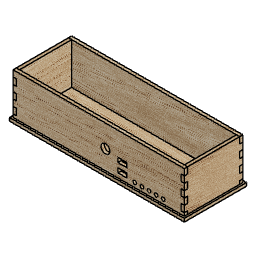
wood chassis (Autodesk Fusion 360 design; units mm, degrees)
Autodesk Fusion 360 part; units mm, degrees
sketch "base" plane through (0, 0, 0) normal (0, 0, 1) x (1, 0, 0) in component "base"
  line L0 (0, 0) -> (192.2, 0)
  line L1 (192.2, 0) -> (192.2, 65.7)
  line L2 (192.2, 65.7) -> (0, 65.7)
  line L3 (0, 65.7) -> (0, 0)
  line L4 (192.2, 32.85) -> (0, 32.85) construction
  line L5 (96.1, 65.7) -> (96.1, 0) construction
  line L6 (-2, 67.7) -> (194.2, 67.7)
  line L7 (194.2, 67.7) -> (194.2, -2)
  line L8 (194.2, -2) -> (-2, -2)
  line L9 (-2, -2) -> (-2, 67.7)
  line L10 (-2, 67.7) -> (194.2, -2) construction
  line L11 (194.2, 67.7) -> (-2, -2) construction
  point P0 (96.1, 32.85)
  dimension "d14" = 192.2
  dimension "d15" = 65.7
  dimension "d16" = 2
  dimension "d17" = 2
  constraint horizontal L0
  constraint vertical L1
  constraint horizontal L2
  constraint vertical L3
  constraint coincident L0.start L3.end
  constraint midpoint L1 L4.start
  constraint midpoint L3 L4.end
  constraint midpoint L2 L5.start
  constraint midpoint L0 L5.end
  constraint horizontal L6
  constraint perpendicular L6 L7
  constraint parallel L6 L8
  constraint parallel L7 L9
  constraint coincident L10 P0
  constraint coincident L11 P0
  constraint midpoint L4 P0
  measures "d14" distance of L1.end L2.end
  measures "d15" distance of L0.end L1.end
  measures "d16" distance of L2 L6
  measures "d17" distance of L1 L7
extrude "Extrude1" add sketch "base" along normal blind 3.6 contours L0 L1 L2 L3 | L6 L7 L8 L9 makes body 1 in component "base"
sketch "lenghttabcut" plane through (0, 0, 3.6) normal (0, 0, 1) x (-1, 0, 0) in component "base"
  line L0 (2, 2) -> (-194.2, 2)
  line L1 (-194.2, 2) -> (-194.2, -67.7)
  line L2 (-194.2, -67.7) -> (2, -67.7)
  line L3 (2, -67.7) -> (2, 2)
  line L4 (-27.4571, -65.7) -> (-54.9143, -65.7)
  line L5 (-54.9143, -65.7) -> (-54.9143, -62.1)
  line L6 (-54.9143, -62.1) -> (-27.4571, -62.1)
  line L7 (-27.4571, -62.1) -> (-27.4571, -65.7)
  line L8 (-192.2, -65.7) -> (0, -65.7)
  line L9 (0, -65.7) -> (0, 0)
  dimension "d20" = 27.4571
  dimension "d21" = 27.4571
  dimension "d35" = 3.6
  constraint horizontal L4
  constraint vertical L5
  constraint horizontal L6
  constraint vertical L7
  constraint collinear L4 L8
  measures "d20" distance of L7 L9
  measures "d21" distance of L4.start L4.end
  measures "d35" distance of L4.start L6.end
extrude "Extrude2" cut sketch "lenghttabcut" against normal blind 3.6 contours L4 L5 L6 L7 L8 bodies 1 in component "base"
pattern_linear "R-Pattern1" count 3 spacing 54.9143 along (1, 0, 0) of "Extrude2" in component "base"
ref_plane "WorkPlane1" through (96.1, 65.7, 1.8) normal (0, 1, 0) x (-1, 0, 0) in component "back"
sketch "back" plane through (30, 65.7, 1.5) normal (0, 1, 0) x (1, 0, 0) in component "back"
  line L0 (-30, 1.5) -> (162.2, 1.5)
  line L1 (162.2, 1.5) -> (162.2, -48.5)
  line L2 (162.2, -48.5) -> (-30, -48.5)
  line L3 (-30, -48.5) -> (-30, 1.5)
  point P0 (66.1, 1.5)
  dimension "d29" = 50
  dimension "d30" = 192.2
  constraint horizontal L0
  constraint vertical L1
  constraint horizontal L2
  constraint vertical L3
  constraint midpoint L0 P0
  measures "d29" distance of L0.start L2.end
  measures "d30" distance of L1.end L2.end
extrude "Extrude1'" add sketch "back" against normal blind 3.6 separate body makes body 2 in component "back"
sketch "heighttabcut" plane through (192.2, 0, 0) normal (1, 0, 0) x (0, 1, 0) in component "back"
  line L0 (65.7, 0) -> (65.7, 50)
  line L1 (65.7, 50) -> (62.1, 50)
  line L2 (62.1, 50) -> (62.1, 0)
  line L3 (62.1, 0) -> (65.7, 0)
  line L4 (62.1, 14.2857) -> (65.7, 14.2857)
  line L5 (65.7, 14.2857) -> (65.7, 7.1429)
  line L6 (65.7, 7.1429) -> (62.1, 7.1429)
  line L7 (62.1, 7.1429) -> (62.1, 14.2857)
  line L8 (67.7, 0) -> (-2, 0)
  dimension "d33" = 7.1429
  dimension "d34" = 7.1429
  constraint horizontal L4
  constraint vertical L5
  constraint horizontal L6
  constraint vertical L7
  constraint coincident L0 L5.end
  constraint coincident L2 L4.start
  measures "d33" distance of L6 L8
  measures "d34" distance of L4.end L5.end
combine "Combine1" operation cut target body 2 tool bodies 1 keep tools in component "back"
extrude "Extrude2'" cut sketch "heighttabcut" against normal blind 3.6 contours L0 L2 L4 L5 L6 L7 bodies 2 in component "back"
pattern_linear "R-Pattern1'" count 3 spacing 14.2857 along (0, 0, 1) of "Extrude2'" in component "back"
extrude "Extrude1''" add 1 faces at (91.5238, 65.7, 34.5333) along direction (0, 1, 0) blind 3.6 from surface at -65.7 separate body on bodies 2 makes body 3 in component "front"
combine "Combine1'" operation cut target body 1 tool bodies 3 keep tools in component "base"
sketch "widthtabcut" plane through (0, 0, 3.6) normal (0, 0, 1) x (-1, 0, 0) in component "base"
  line L0 (-27.4571, 0) -> (-27.4571, -3.6)
  line L1 (-27.4571, -3.6) -> (-54.9143, -3.6)
  line L2 (-54.9143, -3.6) -> (-54.9143, 0)
  line L3 (-54.9143, 0) -> (-27.4571, 0)
  line L4 (-82.3714, 0) -> (-82.3714, -3.6)
  line L5 (-82.3714, -3.6) -> (-109.8286, -3.6)
  line L6 (-109.8286, -3.6) -> (-109.8286, 0)
  line L7 (-109.8286, 0) -> (-82.3714, 0)
  line L8 (-137.2857, 0) -> (-137.2857, -3.6)
  line L9 (-137.2857, -3.6) -> (-164.7429, -3.6)
  line L10 (-164.7429, -3.6) -> (-164.7429, 0)
  line L11 (-164.7429, 0) -> (-137.2857, 0)
  line L12 (-137.2857, -62.1) -> (-137.2857, -65.7)
  line L13 (-137.2857, -65.7) -> (-164.7429, -65.7)
  line L14 (-164.7429, -65.7) -> (-164.7429, -62.1)
  line L15 (-164.7429, -62.1) -> (-137.2857, -62.1)
  line L16 (-82.3714, -62.1) -> (-82.3714, -65.7)
  line L17 (-82.3714, -65.7) -> (-109.8286, -65.7)
  line L18 (-109.8286, -65.7) -> (-109.8286, -62.1)
  line L19 (-109.8286, -62.1) -> (-82.3714, -62.1)
  line L20 (-27.4571, -62.1) -> (-27.4571, -65.7)
  line L21 (-27.4571, -65.7) -> (-54.9143, -65.7)
  line L22 (-54.9143, -65.7) -> (-54.9143, -62.1)
  line L23 (-54.9143, -62.1) -> (-27.4571, -62.1)
  line L24 (2, 2) -> (-194.2, 2)
  line L25 (-194.2, 2) -> (-194.2, -67.7)
  line L26 (-194.2, -67.7) -> (2, -67.7)
  line L27 (2, -67.7) -> (2, 2)
  line L28 (-192.2, -56.3143) -> (-188.6, -56.3143)
  line L29 (-188.6, -56.3143) -> (-188.6, -46.9286)
  line L30 (-188.6, -46.9286) -> (-192.2, -46.9286)
  line L31 (-192.2, -46.9286) -> (-192.2, -56.3143)
  line L32 (-192.2, -65.7) -> (0, -65.7)
  line L33 (-192.2, 0) -> (-192.2, -65.7)
  dimension "d45" = 3.6
  dimension "d46" = 9.3857
  dimension "d47" = 9.3857
  constraint horizontal L28
  constraint vertical L29
  constraint horizontal L30
  constraint vertical L31
  constraint collinear L31 L33
  measures "d45" distance of L28.start L28.end
  measures "d46" distance of L28 L32
  measures "d47" distance of L28.start L30.end
extrude "Extrude3" cut sketch "widthtabcut" against normal blind 3.6 contours L28 L29 L30 L31 L33 bodies 1 in component "base"
pattern_linear "R-Pattern2" count 3 spacing 18.7714 along (0, -1, 0) of "Extrude3" in component "base"
sketch "Sketch1" plane through (192.2, 0, 0) normal (1, 0, 0) x (0, 1, 0) in component "right"
  line L0 (65.7, 42.8571) -> (65.7, 50)
  line L1 (65.7, 50) -> (62.1, 50)
  line L2 (62.1, 50) -> (62.1, 42.8571)
  line L3 (0, 0) -> (65.7, 0)
  line L4 (65.7, 0) -> (65.7, 50)
  line L5 (65.7, 50) -> (0, 50)
  line L6 (0, 50) -> (0, 0)
  line L7 (62.1, 42.8571) -> (65.7, 42.8571)
  constraint perpendicular L3 L4
  constraint parallel L3 L5
  constraint parallel L4 L6
  constraint horizontal L3
  constraint coincident L3.start L6.end
  constraint coincident L0.end L1.start
extrude "Extrude1'''" add sketch "Sketch1" against normal blind 3.6 separate body makes body 4 in component "right"
combine "Combine1''" operation cut target body 4 tool bodies 2 keep tools in component "right"
combine "Combine2" operation cut target body 4 tool bodies 3 keep tools in component "right"
combine "Combine3" operation cut target body 4 tool bodies 1 keep tools in component "right"
extrude "Extrude1''''" add 1 faces at (188.6, 31.2857, 25.0095) along direction (-1, 0, 0) blind 3.6 from surface at 185 separate body on bodies 4 makes body 5 in component "left"
combine "Combine2'" operation cut target body 2 tool bodies 5 keep tools in component "back"
combine "Combine1'''" operation cut target body 3 tool bodies 5 keep tools in component "front"
combine "Combine2''" operation cut target body 1 tool bodies 5 keep tools in component "base"
sketch "chassis cut" plane through (0, 0, 0) normal (0, -1, 0) x (1, 0, 0) in component "front"
  line L0 (3.6, 7.1429) -> (0, 7.1429)
  line L1 (0, 7.1429) -> (0, 3.6)
  line L2 (0, 3.6) -> (27.4571, 3.6)
  line L3 (27.4571, 3.6) -> (27.4571, 0)
  line L4 (27.4571, 0) -> (54.9143, 0)
  line L5 (54.9143, 0) -> (54.9143, 3.6)
  line L6 (54.9143, 3.6) -> (82.3714, 3.6)
  line L7 (82.3714, 3.6) -> (82.3714, 0)
  line L8 (82.3714, 0) -> (109.8286, 0)
  line L9 (109.8286, 0) -> (109.8286, 3.6)
  line L10 (109.8286, 3.6) -> (137.2857, 3.6)
  line L11 (137.2857, 3.6) -> (137.2857, 0)
  line L12 (137.2857, 0) -> (164.7429, 0)
  line L13 (164.7429, 0) -> (164.7429, 3.6)
  line L14 (164.7429, 3.6) -> (192.2, 3.6)
  line L15 (192.2, 3.6) -> (192.2, 7.1429)
  line L16 (192.2, 7.1429) -> (188.6, 7.1429)
  line L17 (188.6, 7.1429) -> (188.6, 14.2857)
  line L18 (188.6, 14.2857) -> (192.2, 14.2857)
  line L19 (192.2, 14.2857) -> (192.2, 21.4286)
  line L20 (192.2, 21.4286) -> (188.6, 21.4286)
  line L21 (188.6, 21.4286) -> (188.6, 28.5714)
  line L22 (188.6, 28.5714) -> (192.2, 28.5714)
  line L23 (192.2, 28.5714) -> (192.2, 35.7143)
  line L24 (192.2, 35.7143) -> (188.6, 35.7143)
  line L25 (188.6, 35.7143) -> (188.6, 42.8571)
  line L26 (188.6, 42.8571) -> (192.2, 42.8571)
  line L27 (192.2, 42.8571) -> (192.2, 50)
  line L28 (192.2, 50) -> (0, 50)
  line L29 (0, 50) -> (0, 42.8571)
  line L30 (0, 42.8571) -> (3.6, 42.8571)
  line L31 (3.6, 42.8571) -> (3.6, 35.7143)
  line L32 (3.6, 35.7143) -> (0, 35.7143)
  line L33 (0, 35.7143) -> (0, 28.5714)
  line L34 (0, 28.5714) -> (3.6, 28.5714)
  line L35 (3.6, 28.5714) -> (3.6, 21.4286)
  line L36 (3.6, 21.4286) -> (0, 21.4286)
  line L37 (0, 21.4286) -> (0, 14.2857)
  line L38 (0, 14.2857) -> (3.6, 14.2857)
  line L39 (3.6, 14.2857) -> (3.6, 7.1429)
  circle A0 centre (103.6, 25) radius 5
  line L40 (117.6, 13.6) -> (127.6, 13.6)
  line L41 (127.6, 13.6) -> (127.6, 8.6)
  line L42 (127.6, 8.6) -> (117.6, 8.6)
  line L43 (117.6, 8.6) -> (117.6, 13.6)
  line L44 (117.6, 13.6) -> (127.6, 8.6) construction
  line L45 (127.6, 13.6) -> (117.6, 8.6) construction
  line L46 (117.6, 23.6) -> (127.6, 23.6)
  line L47 (127.6, 23.6) -> (127.6, 18.6)
  line L48 (127.6, 18.6) -> (117.6, 18.6)
  line L49 (117.6, 18.6) -> (117.6, 23.6)
  line L50 (117.6, 23.6) -> (127.6, 18.6) construction
  line L51 (127.6, 23.6) -> (117.6, 18.6) construction
  circle A1 centre (136.6, 8.6) radius 2
  circle A2 centre (152.6, 8.6) radius 2
  circle A3 centre (144.6, 8.6) radius 2
  circle A4 centre (160.6, 8.6) radius 2
  circle A5 centre (168.6, 8.6) radius 2
  line L52 (169.5326, 10.6) -> (169.1044, 10.6)
  line L53 (169.1044, 10.6) -> (134.2723, 10.6) construction
  line L54 (-2, 3.6) -> (194.2, 3.6)
  point P0 (122.6, 11.1)
  point P1 (122.6, 21.1)
  dimension "d59" = 10
  dimension "d60" = 25
  dimension "d61" = 100
  dimension "d62" = 10
  dimension "d63" = 5
  dimension "d64" = 5
  dimension "d68" = 4
  dimension "d69" = 8
  dimension "d70" = 8
  dimension "d71" = 8
  dimension "d72" = 8
  dimension "d74" = 5
  dimension "d75" = 20
  constraint horizontal L40
  constraint perpendicular L40 L41
  constraint parallel L40 L42
  constraint parallel L41 L43
  constraint coincident L44 P0
  constraint coincident L45 P0
  constraint horizontal L46
  constraint perpendicular L46 L47
  constraint parallel L46 L48
  constraint parallel L47 L49
  constraint coincident L50 P1
  constraint coincident L51 P1
  constraint collinear L41 L47
  constraint collinear L43 L49
  constraint equal L41 L47
  constraint equal A4 A5
  constraint equal A3 A4
  constraint equal A2 A3
  constraint equal A1 A2
  constraint horizontal L52
  constraint parallel L52 L53
  constraint tangent A5 L53
  constraint tangent A4 L53
  constraint tangent A2 L53
  constraint tangent A3 L53
  constraint tangent A1 L53
  measures "d59" diameter of A0
  measures "d60" distance of L28 A0.centre
  measures "d61" distance of L31 A0.centre
  measures "d62" distance of L46.start L46.end
  measures "d63" distance of L46.start L48.end
  measures "d64" distance of L40 L48
  measures "d68" diameter of A3
  measures "d69" distance of A1.centre A3.centre
  measures "d70" distance of A2.centre A3.centre
  measures "d71" distance of A2.centre A4.centre
  measures "d72" distance of A4.centre A5.centre
  measures "d74" distance of A4.centre L54
  measures "d75" distance of L17 A5.centre
extrude "Extrude2''" cut sketch "chassis cut" against normal blind 3.6 contours A0 | L40 L41 L42 L43 | L46 L47 L48 L49 | A1 | A2 | A3 | A4 | A5 bodies 3 in component "front"
component "base" placed x (1, 0, 0) y (0, 1, 0) z (0, 0, 1) at (0, 0, 0)
component "back" placed x (1, 0, 0) y (0, 1, 0) z (0, 0, 1) at (0, 0, 0)
component "front" placed x (1, 0, 0) y (0, 1, 0) z (0, 0, 1) at (0, 0, 0)
component "right" placed x (1, 0, 0) y (0, 1, 0) z (0, 0, 1) at (0, 0, 0)
component "left" placed x (1, 0, 0) y (0, 1, 0) z (0, 0, 1) at (0, 0, 0)
equation "length = 185 mm + thick * 2" comment "exterior"
equation "width = 58.5 mm + thick * 2" comment "exterior"
equation "height = 50 mm" comment "exterior"
equation "thick = 3.6 mm" comment "material thickness"
equation "Ltab = 3" comment "No. tab"
equation "Wtab = 3" comment "No. tab"
equation "Htab = 3" comment "No. tab"
equation "WtabWidth = width / ( ( Wtab * 2 ) + 1 )" comment "tab size"
equation "LtabWidth = length / ( ( Ltab * 2 ) + 1 )" comment "tab size"
equation "HtabWidth = height / ( ( Htab * 2 ) + 1 )" comment "tab size"
equation "baseoffset = 2 mm" comment "Base outline"
equation "d14 = length"
equation "d15 = width"
equation "d16 = baseoffset"
equation "d17 = baseoffset"
equation "d18 = thick"
equation "d20 = LtabWidth"
equation "d21 = LtabWidth"
equation "d22 = -thick"
equation "d24 = Ltab"
equation "d26 = length - LtabWidth * 3"
equation "d28 = -baseoffset"
equation "d29 = height"
equation "d30 = length"
equation "d31 = -thick"
equation "d33 = HtabWidth"
equation "d34 = HtabWidth"
equation "d35 = thick"
equation "d36 = -thick"
equation "d38 = Htab"
equation "d40 = height - HtabWidth * 3"
equation "d42 = -baseoffset"
equation "d43 = thick"
equation "d45 = thick"
equation "d46 = WtabWidth"
equation "d47 = WtabWidth"
equation "d48 = -thick"
equation "d50 = Wtab"
equation "d52 = width - WtabWidth * 3"
equation "d54 = -thick"
equation "d56 = -baseoffset - thick"
equation "d57 = thick"
equation "d76 = -thick"
